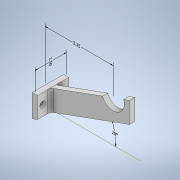
# Autodesk Inventor part: PipeSupport-3_25-020
Saved by Autodesk Inventor 2021.1 (Build 251245010, 245A)
## iProperties
Created: 2020-09-15
Part Number: PipeSupport-3_25-020
Material: Generic
Document SubType Name: Modeling
Designer: robst
Density: 1 g/cm^3
Appearance: Default
Author: robst
Autodesk Inventor part; units mm, degrees
ref_plane "YZ Plane" through (0, 0, 0) normal (1, 0, 0) x (0, 1, 0)
ref_plane "XZ Plane" through (0, 0, 0) normal (0, 1, 0) x (-1, 0, 0)
ref_plane "XY Plane" through (0, 0, 0) normal (0, 0, 1) x (1, 0, 0)
sketch "Sketch5" plane through (0, 0, 0) normal (0, 0, 1) x (1, 0, 0)
  line L0 (0, 0) -> (6.35, 0)
  line L1 (6.35, 0) -> (6.35, 25.4)
  line L2 (6.35, 25.4) -> (0, 25.4)
  line L3 (0, 25.4) -> (0, 0)
  dimension "d21" = 25.4
  dimension "d22" = 6.35
  constraints: 8 end point, 2 parallel, 1 horizontal, 1 perpendicular
  measures "d21" distance from line of L2 L0.start
  measures "d22" distance from line of L1 L0.start
extrude "Extrusion3" add sketch "Sketch5" against normal mid plane 38.1
sketch "Sketch6" plane through (0, 0, 0) normal (0, 0, 1) x (1, 0, 0)
  line L0 (6.35, 25.4) -> (6.35, 0) projected
  line L1 (0, 25.4) -> (6.35, 25.4) projected
  line L2 (6.35, 0) -> (0, 0) projected
  line L3 (0, 0) -> (0, 25.4) projected
  line L4 (6.35, 0) -> (102.5525, 35.0148)
  line L5 (6.35, 0) -> (108.7266, 0) construction
  line L6 (102.5525, 60.4148) -> (102.5525, 35.0148)
  arc A0 (69.7208, 48.4651) -> (95.3792, 57.804) centre (82.55, 53.1345) ccw
  line L7 (6.35, 25.4) -> (69.7208, 48.4651)
  line L8 (95.3792, 57.804) -> (102.5525, 60.4148)
  dimension "d25" = 20
  dimension "d26" = 27.305
  dimension "d29" = 6.35
  dimension "d30" = 82.55
  dimension "d33" = 0
  constraints: 10 end point, 2 parallel, 2 point on circle, 1 centre point, 1 collinear, 1 equal length, 1 horizontal, 1 vertical
  measures "d25" angle of L5 L4
  measures "d26" diameter of A0
  measures "d29" distance edge to line of A0 L6
  measures "d30" distance from line of A0.centre L3
  measures "d33" distance from line of L7 A0.centre
extrude "Extrusion4" add sketch "Sketch6" along normal mid plane 6.35 contours L7 A0 L8 L6 L4 L0
sketch "Sketch7" plane through (6.35, 0, 19.05) normal (1, 0, 0) x (0, 0, -1)
  line L0 (38.1, 25.4) -> (0, 25.4) construction
  line L1 (6.35, 25.4) -> (6.35, 0) construction
  line L2 (31.75, 25.4) -> (31.75, 0) construction
  line L3 (0, 0) -> (0, 25.4) construction
  line L4 (38.1, 25.4) -> (38.1, 0) construction
  line L5 (0, 0) -> (15.875, 0) projected
  line L6 (22.225, 0) -> (38.1, 0) projected
  point P0 (19.05, 0)
  point P1 (6.35, 12.7)
  point P2 (31.75, 12.7)
  dimension "d34" = 6.35
  dimension "d35" = 6.35
  constraints: 4 end point, 2 midpoint, 2 point on line, 2 vertical
  measures "d34" distance between parallel lines of L1 L3
  measures "d35" distance between parallel lines of L2 L4
sketch "Sketch8" plane through (0, 0, 0) normal (0, 0, 1) x (1, 0, 0)
  line L0 (0, 0) -> (0, 25.4) projected
  line L1 (6.35, 0) -> (0, 0) projected
  line L2 (102.5525, 35.0148) -> (6.35, 0) projected
  line L3 (0, 0) -> (6.35, 0)
  line L4 (0, -2.3112) -> (6.35, 0)
  line L5 (0, 0) -> (0, -2.3112)
  constraints: 6 end point, 2 collinear, 1 vertical
extrude "Extrusion5" add sketch "Sketch8" along normal mid plane 38.1
hole "Hole3" at (6.35, 12.7, 12.7) at (6.35, 12.7, -12.7) direction (-1, 0, 0) diameter 3.81 end through all countersink diameter 7.0866 countersink angle 82 clearance for "Flat Head Machine Screw (82)" size "#6" standard "Ansi Unified Screw Threads"
sketch "Sketch9" plane through (0, 25.4, -19.05) normal (-1, 0, 0) x (0, 0, 1)
  line L0 (0, -27.7112) -> (0, 0) projected
  line L1 (38.1, 0) -> (38.1, -27.7112) projected
  line L2 (0, 0) -> (0, -25.4) construction
  line L3 (0, -13.8556) -> (38.1, -13.8556) construction
  spline S0 degree 2 poles (11.2596, -12.6206) (11.1484, -12.6206) (10.9286, -12.6749) (10.8224, -12.7169) knots 0 0 0 1 2 2 2
  spline S1 degree 2 poles (10.8224, -12.7169) (10.7236, -12.7589) (10.5778, -12.8478) (10.521, -12.8874) knots 0 0 0 1 2 2 2
  line L4 (10.521, -12.8874) -> (10.4963, -12.8874)
  line L5 (10.4963, -12.8874) -> (10.4963, -12.4551)
  spline S2 degree 2 poles (10.4963, -12.4551) (10.6297, -12.3835) (11.0867, -12.2674) (11.2917, -12.2674) knots 0 0 0 1 2 2 2
  spline S3 degree 2 poles (11.2917, -12.2674) (11.4992, -12.2674) (11.8079, -12.3514) (11.9339, -12.4403) knots 0 0 0 1 2 2 2
  spline S4 degree 2 poles (11.9339, -12.4403) (12.0673, -12.5366) (12.2056, -12.8157) (12.2056, -13.0034) knots 0 0 0 1 2 2 2
  spline S5 degree 2 poles (12.2056, -13.0034) (12.2056, -13.2554) (11.8746, -13.6358) (11.6424, -13.6852) knots 0 0 0 1 2 2 2
  line L6 (11.6424, -13.6852) -> (11.6424, -13.7148)
  spline S6 degree 2 poles (11.6424, -13.7148) (11.7388, -13.7346) (11.9586, -13.8235) (12.0524, -13.9124) knots 0 0 0 1 2 2 2
  spline S7 degree 2 poles (12.0524, -13.9124) (12.1463, -13.9989) (12.2649, -14.2755) (12.2649, -14.4756) knots 0 0 0 1 2 2 2
  spline S8 degree 2 poles (12.2649, -14.4756) (12.2649, -14.6806) (12.1241, -15.0289) (11.9956, -15.1622) knots 0 0 0 1 2 2 2
  spline S9 degree 2 poles (11.9956, -15.1622) (11.8623, -15.3006) (11.4843, -15.4438) (11.2447, -15.4438) knots 0 0 0 1 2 2 2
  spline S10 degree 2 poles (11.2447, -15.4438) (11.015, -15.4438) (10.5655, -15.3327) (10.4124, -15.2561) knots 0 0 0 1 2 2 2
  line L7 (10.4124, -15.2561) -> (10.4124, -14.8239)
  line L8 (10.4124, -14.8239) -> (10.442, -14.8239)
  spline S11 degree 2 poles (10.442, -14.8239) (10.5704, -14.9177) (11.0052, -15.0906) (11.22, -15.0906) knots 0 0 0 1 2 2 2
  spline S12 degree 2 poles (11.22, -15.0906) (11.346, -15.0906) (11.598, -15.0116) (11.6819, -14.9202) knots 0 0 0 1 2 2 2
  spline S13 degree 2 poles (11.6819, -14.9202) (11.7635, -14.8288) (11.8499, -14.6114) (11.8499, -14.4459) knots 0 0 0 1 2 2 2
  spline S14 degree 2 poles (11.8499, -14.4459) (11.8499, -14.2804) (11.7536, -14.0656) (11.6671, -14.0038) knots 0 0 0 1 2 2 2
  spline S15 degree 2 poles (11.6671, -14.0038) (11.5807, -13.9421) (11.346, -13.8951) (11.2077, -13.8951) knots 0 0 0 1 2 2 2
  line L9 (11.2077, -13.8951) -> (11.0348, -13.8951)
  line L10 (11.0348, -13.8951) -> (11.0348, -13.5567)
  line L11 (11.0348, -13.5567) -> (11.1706, -13.5567)
  spline S16 degree 2 poles (11.1706, -13.5567) (11.4448, -13.5567) (11.7906, -13.2949) (11.7906, -13.0454) knots 0 0 0 1 2 2 2
  spline S17 degree 2 poles (11.7906, -13.0454) (11.7906, -12.9293) (11.7017, -12.7639) (11.6301, -12.7145) knots 0 0 0 1 2 2 2
  spline S18 degree 2 poles (11.6301, -12.7145) (11.5535, -12.6626) (11.3658, -12.6206) (11.2596, -12.6206) knots 0 0 0 1 2 2 2
  line L12 (13.3788, -15.3796) -> (12.8898, -15.3796)
  line L13 (12.8898, -15.3796) -> (12.8898, -14.7967)
  line L14 (12.8898, -14.7967) -> (13.3788, -14.7967)
  line L15 (13.3788, -14.7967) -> (13.3788, -15.3796)
  line L16 (15.8736, -15.3796) -> (13.9939, -15.3796)
  line L17 (13.9939, -15.3796) -> (13.9939, -14.9474)
  spline S19 degree 2 poles (13.9939, -14.9474) (14.1964, -14.7572) (14.557, -14.4039) (14.7299, -14.2138) knots 0 0 0 1 2 2 2
  spline S20 degree 2 poles (14.7299, -14.2138) (15.0782, -13.8309) (15.3326, -13.3715) (15.3326, -13.127) knots 0 0 0 1 2 2 2
  spline S21 degree 2 poles (15.3326, -13.127) (15.3326, -12.9985) (15.2536, -12.8058) (15.182, -12.7441) knots 0 0 0 1 2 2 2
  spline S22 degree 2 poles (15.182, -12.7441) (15.1103, -12.6823) (14.9226, -12.6206) (14.809, -12.6206) knots 0 0 0 1 2 2 2
  spline S23 degree 2 poles (14.809, -12.6206) (14.7003, -12.6206) (14.478, -12.6749) (14.3767, -12.7169) knots 0 0 0 1 2 2 2
  spline S24 degree 2 poles (14.3767, -12.7169) (14.2903, -12.7515) (14.1297, -12.8503) (14.0803, -12.8849) knots 0 0 0 1 2 2 2
  line L18 (14.0803, -12.8849) -> (14.0581, -12.8849)
  line L19 (14.0581, -12.8849) -> (14.0581, -12.4502)
  spline S25 degree 2 poles (14.0581, -12.4502) (14.1841, -12.3884) (14.6361, -12.2674) (14.8386, -12.2674) knots 0 0 0 1 2 2 2
  spline S26 degree 2 poles (14.8386, -12.2674) (15.2659, -12.2674) (15.7476, -12.7194) (15.7476, -13.1047) knots 0 0 0 1 2 2 2
  spline S27 degree 2 poles (15.7476, -13.1047) (15.7476, -13.285) (15.6636, -13.5864) (15.5895, -13.7148) knots 0 0 0 1 2 2 2
  spline S28 degree 2 poles (15.5895, -13.7148) (15.5154, -13.8482) (15.3005, -14.11) (15.182, -14.236) knots 0 0 0 1 2 2 2
  spline S29 degree 2 poles (15.182, -14.236) (14.9893, -14.4459) (14.5175, -14.8955) (14.3767, -15.0264) knots 0 0 0 1 2 2 2
  line L20 (14.3767, -15.0264) -> (15.8736, -15.0264)
  line L21 (15.8736, -15.0264) -> (15.8736, -15.3796)
  spline S30 degree 2 poles (18.1287, -14.4114) (18.1287, -14.6312) (17.9879, -15.0066) (17.8595, -15.145) knots 0 0 0 1 2 2 2
  spline S31 degree 2 poles (17.8595, -15.145) (17.731, -15.2833) (17.3482, -15.4438) (17.111, -15.4438) knots 0 0 0 1 2 2 2
  spline S32 degree 2 poles (17.111, -15.4438) (16.8937, -15.4438) (16.4688, -15.3475) (16.3132, -15.2709) knots 0 0 0 1 2 2 2
  line L22 (16.3132, -15.2709) -> (16.3132, -14.8387)
  line L23 (16.3132, -14.8387) -> (16.3429, -14.8387)
  spline S33 degree 2 poles (16.3429, -14.8387) (16.3898, -14.8733) (16.5652, -14.9622) (16.6714, -15.0017) knots 0 0 0 1 2 2 2
  spline S34 degree 2 poles (16.6714, -15.0017) (16.7924, -15.0437) (16.9925, -15.0906) (17.1184, -15.0906) knots 0 0 0 1 2 2 2
  spline S35 degree 2 poles (17.1184, -15.0906) (17.2419, -15.0906) (17.4741, -15.0017) (17.5581, -14.9054) knots 0 0 0 1 2 2 2
  spline S36 degree 2 poles (17.5581, -14.9054) (17.6347, -14.814) (17.7137, -14.5719) (17.7137, -14.4089) knots 0 0 0 1 2 2 2
  spline S37 degree 2 poles (17.7137, -14.4089) (17.7137, -14.2459) (17.6248, -14.0384) (17.5408, -13.9692) knots 0 0 0 1 2 2 2
  spline S38 degree 2 poles (17.5408, -13.9692) (17.4544, -13.8927) (17.1975, -13.8284) (17.0419, -13.8284) knots 0 0 0 1 2 2 2
  spline S39 degree 2 poles (17.0419, -13.8284) (16.8739, -13.8284) (16.5405, -13.8803) (16.4392, -13.9025) knots 0 0 0 1 2 2 2
  line L24 (16.4392, -13.9025) -> (16.4392, -12.3316)
  line L25 (16.4392, -12.3316) -> (18.1114, -12.3316)
  line L26 (18.1114, -12.3316) -> (18.1114, -12.6898)
  line L27 (18.1114, -12.6898) -> (16.8319, -12.6898)
  line L28 (16.8319, -12.6898) -> (16.8319, -13.5024)
  spline S40 degree 2 poles (16.8319, -13.5024) (16.906, -13.4925) (17.0493, -13.4851) (17.1086, -13.4851) knots 0 0 0 1 2 2 2
  spline S41 degree 2 poles (17.1086, -13.4851) (17.3432, -13.4851) (17.6668, -13.5617) (17.815, -13.6753) knots 0 0 0 1 2 2 2
  spline S42 degree 2 poles (17.815, -13.6753) (17.9657, -13.7889) (18.1287, -14.1347) (18.1287, -14.4114) knots 0 0 0 1 2 2 2
  line L29 (19.0253, -12.1958) -> (18.9364, -13.3814)
  line L30 (18.9364, -13.3814) -> (18.6671, -13.3814)
  line L31 (18.6671, -13.3814) -> (18.5782, -12.1958)
  line L32 (18.5782, -12.1958) -> (19.0253, -12.1958)
  line L33 (19.7959, -12.1958) -> (19.707, -13.3814)
  line L34 (19.707, -13.3814) -> (19.4378, -13.3814)
  line L35 (19.4378, -13.3814) -> (19.3489, -12.1958)
  line L36 (19.3489, -12.1958) -> (19.7959, -12.1958)
  line L37 (23.4392, -15.3796) -> (21.5595, -15.3796)
  line L38 (21.5595, -15.3796) -> (21.5595, -14.9474)
  spline S43 degree 2 poles (21.5595, -14.9474) (21.7621, -14.7572) (22.1227, -14.4039) (22.2956, -14.2138) knots 0 0 0 1 2 2 2
  spline S44 degree 2 poles (22.2956, -14.2138) (22.6439, -13.8309) (22.8983, -13.3715) (22.8983, -13.127) knots 0 0 0 1 2 2 2
  spline S45 degree 2 poles (22.8983, -13.127) (22.8983, -12.9985) (22.8192, -12.8058) (22.7476, -12.7441) knots 0 0 0 1 2 2 2
  spline S46 degree 2 poles (22.7476, -12.7441) (22.676, -12.6823) (22.4883, -12.6206) (22.3746, -12.6206) knots 0 0 0 1 2 2 2
  spline S47 degree 2 poles (22.3746, -12.6206) (22.266, -12.6206) (22.0437, -12.6749) (21.9424, -12.7169) knots 0 0 0 1 2 2 2
  spline S48 degree 2 poles (21.9424, -12.7169) (21.8559, -12.7515) (21.6954, -12.8503) (21.646, -12.8849) knots 0 0 0 1 2 2 2
  line L39 (21.646, -12.8849) -> (21.6238, -12.8849)
  line L40 (21.6238, -12.8849) -> (21.6238, -12.4502)
  spline S49 degree 2 poles (21.6238, -12.4502) (21.7497, -12.3884) (22.2017, -12.2674) (22.4043, -12.2674) knots 0 0 0 1 2 2 2
  spline S50 degree 2 poles (22.4043, -12.2674) (22.8316, -12.2674) (23.3132, -12.7194) (23.3132, -13.1047) knots 0 0 0 1 2 2 2
  spline S51 degree 2 poles (23.3132, -13.1047) (23.3132, -13.285) (23.2293, -13.5864) (23.1552, -13.7148) knots 0 0 0 1 2 2 2
  spline S52 degree 2 poles (23.1552, -13.7148) (23.0811, -13.8482) (22.8662, -14.11) (22.7476, -14.236) knots 0 0 0 1 2 2 2
  spline S53 degree 2 poles (22.7476, -14.236) (22.555, -14.4459) (22.0832, -14.8955) (21.9424, -15.0264) knots 0 0 0 1 2 2 2
  line L41 (21.9424, -15.0264) -> (23.4392, -15.0264)
  line L42 (23.4392, -15.0264) -> (23.4392, -15.3796)
  spline S54 degree 2 poles (25.7437, -13.8556) (25.7437, -14.6757) (25.267, -15.4438) (24.7706, -15.4438) knots 0 0 0 1 2 2 2
  spline S55 degree 2 poles (24.7706, -15.4438) (24.2667, -15.4438) (23.7949, -14.6608) (23.7949, -13.8581) knots 0 0 0 1 2 2 2
  spline S56 degree 2 poles (23.7949, -13.8581) (23.7949, -13.0331) (24.2716, -12.2699) (24.7706, -12.2699) knots 0 0 0 1 2 2 2
  spline S57 degree 2 poles (24.7706, -12.2699) (25.272, -12.2699) (25.7437, -13.0603) (25.7437, -13.8556) knots 0 0 0 1 2 2 2
  spline S58 degree 2 poles (25.2201, -14.7843) (25.2794, -14.6337) (25.3288, -14.1693) (25.3288, -13.8556) knots 0 0 0 1 2 2 2
  spline S59 degree 2 poles (25.3288, -13.8556) (25.3288, -13.5419) (25.2794, -13.08) (25.2176, -12.9244) knots 0 0 0 1 2 2 2
  spline S60 degree 2 poles (25.2176, -12.9244) (25.1559, -12.7688) (24.941, -12.6082) (24.7706, -12.6082) knots 0 0 0 1 2 2 2
  spline S61 degree 2 poles (24.7706, -12.6082) (24.6001, -12.6082) (24.3803, -12.7688) (24.3161, -12.9293) knots 0 0 0 1 2 2 2
  spline S62 degree 2 poles (24.3161, -12.9293) (24.2543, -13.085) (24.2099, -13.5592) (24.2099, -13.8581) knots 0 0 0 1 2 2 2
  spline S63 degree 2 poles (24.2099, -13.8581) (24.2099, -14.1792) (24.2494, -14.609) (24.3136, -14.7769) knots 0 0 0 1 2 2 2
  spline S64 degree 2 poles (24.3136, -14.7769) (24.3729, -14.935) (24.5927, -15.1054) (24.7706, -15.1054) knots 0 0 0 1 2 2 2
  spline S65 degree 2 poles (24.7706, -15.1054) (24.9385, -15.1054) (25.1584, -14.9449) (25.2201, -14.7843) knots 0 0 0 1 2 2 2
  spline S66 degree 2 poles (27.6778, -13.0578) (27.6778, -13.3863) (27.2282, -13.8358) (26.8997, -13.8358) knots 0 0 0 1 2 2 2
  spline S67 degree 2 poles (26.8997, -13.8358) (26.5737, -13.8358) (26.1192, -13.3888) (26.1192, -13.0578) knots 0 0 0 1 2 2 2
  spline S68 degree 2 poles (26.1192, -13.0578) (26.1192, -12.7293) (26.5687, -12.2797) (26.8997, -12.2797) knots 0 0 0 1 2 2 2
  spline S69 degree 2 poles (26.8997, -12.2797) (27.2282, -12.2797) (27.6778, -12.7293) (27.6778, -13.0578) knots 0 0 0 1 2 2 2
  spline S70 degree 2 poles (27.3567, -13.0578) (27.3567, -12.8602) (27.0948, -12.591) (26.8997, -12.591) knots 0 0 0 1 2 2 2
  spline S71 degree 2 poles (26.8997, -12.591) (26.7021, -12.591) (26.4403, -12.8602) (26.4403, -13.0578) knots 0 0 0 1 2 2 2
  spline S72 degree 2 poles (26.4403, -13.0578) (26.4403, -13.2579) (26.7071, -13.5246) (26.8997, -13.5246) knots 0 0 0 1 2 2 2
  spline S73 degree 2 poles (26.8997, -13.5246) (27.0948, -13.5246) (27.3567, -13.2529) (27.3567, -13.0578) knots 0 0 0 1 2 2 2
  point P0 (19.05, -25.4)
  constraints: 2 end point, 1 horizontal, 1 midpoint, 1 point on line
extrude "Extrusion6" cut sketch "Sketch9" against normal blind 1.27
fillet "Fillet1" radius 3.175 2 edges at (6.35, 12.7, 3.175) (6.35, 12.7, -3.175)
equation "\"d21\" = supportHeight"
equation "\"d22\" = supportWidth"
equation "\"d23\" = totalScrewHoldWidth"
equation "\"d25\" = supportAngle"
equation "\"d26\" = pipeDiameter"
equation "\"d30\" = distanceFromWallToPipeCenter"
equation "\"d31\" = supportWidth"
equation "\"d34\" = distanceFromEdgeToHoleCenters"
equation "\"d35\" = distanceFromEdgeToHoleCenters"
equation "\"d47\" = totalScrewHoldWidth"
equation "\"pipeDiameter\" = 27.305"
equation "\"distanceFromWallToPipeCenter\" = 82.55"
equation "\"supportHeight\" = 25.4"
equation "\"supportWidth\" = 6.35"
equation "\"screwHoldDepth\" = 6.35"
equation "\"totalScrewHoldWidth\" = 38.1"
equation "\"screwPositionFromTop\" = 6.35"
equation "\"supportAngle\" = 20deg"
equation "\"distanceFromEdgeToHoleCenters\" = 6.35"
body "Solid1"
body "Solid2"
